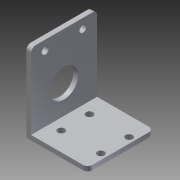
# Autodesk Inventor part: Angle Aluminum P60 Mount
Saved by Autodesk Inventor 2013 (Build 170138000, 138)
## iProperties
Created: 2013-03-11
Part Number: Angle Aluminum P60 Mount
Material: Aluminum 6061
Document SubType Name: Modeling
Designer: Moses
Mass: 27.796 g
Surface Area: 73.4229 cm^2
Volume: 10.2568 cm^3
Density: 2.71 g/cm^3
Author: Moses
Autodesk Inventor part; units mm, degrees
ref_plane "YZ Plane" through (0, 0, 0) normal (1, 0, 0) x (0, 1, 0)
ref_plane "XZ Plane" through (0, 0, 0) normal (0, 1, 0) x (-1, 0, 0)
ref_plane "XY Plane" through (0, 0, 0) normal (0, 0, 1) x (1, 0, 0)
sketch "Sketch1" plane through (0, 0, 0) normal (0, 0, 1) x (1, 0, 0)
  line L0 (0, 0) -> (50.8, 0)
  line L1 (0, 0) -> (0, 63.5)
  line L2 (0, 63.5) -> (3.175, 63.5)
  line L3 (3.175, 63.5) -> (3.175, 3.175)
  line L4 (3.175, 3.175) -> (50.8, 3.175)
  line L5 (50.8, 3.175) -> (50.8, 0)
  dimension "d0" = 50.8
  dimension "d1" = 63.5
  dimension "d2" = 3.175
  constraints: 12 end point, 4 perpendicular, 2 parallel, 1 horizontal
  measures "d0" distance of L0.start L0.end
  measures "d1" distance of L0.start L1.end
  measures "d2" distance of L1.end L2.end
extrude "Extrusion1" add sketch "Sketch1" along normal blind 44.45
sketch "Sketch2" plane through (0, 0, 0) normal (-1, 0, 0) x (0, 0, 1)
  line L0 (0, 0) -> (44.45, 0) projected
  line L1 (0, 63.5) -> (44.45, 63.5) projected
  line L2 (22.225, 63.5) -> (22.225, 0) construction
  line L3 (9.525, 47.625) -> (34.925, 47.625) construction
  circle A0 centre (9.525, 47.625) radius 2.3812
  circle A1 centre (34.925, 47.625) radius 2.3813
  circle A2 centre (22.225, 22.225) radius 9.525
  line L4 (0, 63.5) -> (0, 0) projected
  line L5 (44.45, 63.5) -> (44.45, 0) projected
  line L6 (0, 53.975) -> (44.45, 53.975)
  point P0 (22.225, 47.625)
  dimension "d5" = 25.4
  dimension "d6" = 15.875
  dimension "d7" = 4.7625
  dimension "d8" = 4.7625
  dimension "d11" = 19.05
  dimension "d12" = 22.225
  dimension "d30" = 9.525
  constraints: 6 end point, 4 point on line, 3 centre point, 3 midpoint, 2 coincident, 2 perpendicular
  measures "d5" distance of L3.start L3.end
  measures "d6" distance between parallel lines of L3 L1
  measures "d7" diameter of A0
  measures "d8" diameter of A1
  measures "d11" diameter of A2
  measures "d12" distance from line of L0 A2.centre
  measures "d30" distance between parallel lines of L1 L6
extrude "Extrusion2" cut sketch "Sketch2" against normal blind 38.1 contours L4 L1 L5 L6 | A0 | A1 | A2
sketch "Sketch3" plane through (0, 0, 0) normal (0, -1, 0) x (1, 0, 0)
  line L0 (50.8, 0) -> (50.8, 44.45) projected
  line L1 (0, 0) -> (0, 44.45) projected
  circle A0 centre (10.795, 31.75) radius 2.3813
  line L2 (10.795, 31.75) -> (10.795, 12.7) construction
  circle A1 centre (10.795, 12.7) radius 2.3813
  line L3 (0, 22.225) -> (50.8, 22.225) construction
  line L4 (0, 0) -> (50.8, 0) projected
  line L5 (0, 44.45) -> (50.8, 44.45) projected
  line L6 (41.275, 44.45) -> (41.275, 0)
  circle A2 centre (37.465, 31.75) radius 2.3813
  circle A3 centre (37.465, 12.7) radius 2.3813
  point P0 (10.795, 22.225)
  dimension "d13" = 19.05
  dimension "d17" = 4.7625
  dimension "d18" = 10.795
  dimension "d21" = 41.275
  dimension "d24" = 26.67
  constraints: 6 end point, 4 centre point, 3 midpoint, 3 point on line, 1 coincident, 1 equal radius, 1 horizontal, 1 parallel, 1 perpendicular, 4 other
  measures "d13" distance of L2.start L2.end
  measures "d17" diameter of A0
  measures "d18" distance between parallel lines of L2 L1
  measures "d21" distance between parallel lines of L1 L6
  measures "d24" distance of L2.start A2.centre
extrude "Extrusion3" cut sketch "Sketch3" against normal blind 25.4 contours L4 L6 L5 L0 | A0 | A1 | A2 | A3
fillet "Fillet1" radius 3.175 4 edges at (41.275, 1.5875, 44.45) (41.275, 1.5875, 0) (1.5875, 53.975, 44.45) (1.5875, 53.975, 0)
body "Solid1"
